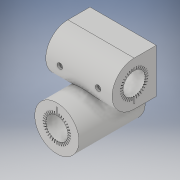
# Autodesk Inventor part: cam_holder_angle_part
Saved by Autodesk Inventor 2019 (Build 230136000, 136)
## iProperties
Created: 2024-08-06
Part Number: cam_holder_angle_part
Material: Generisch
Document SubType Name: Modeling
Designer: nic
Density: 1 g/cm^3
Appearance: Vorgabe
Author: nic
Autodesk Inventor part; units mm, degrees
ref_plane "YZ Plane" through (0, 0, 0) normal (1, 0, 0) x (0, 1, 0)
sketch "Skizze1" plane through (0, 0, 0) normal (0, 0, 1) x (1, 0, 0)
  circle A0 centre (0, 0) radius 10.05
  circle A1 centre (0, 0) radius 20
  dimension "d0" = 20.1
  dimension "d1" = 40
  constraints: 2 centre point, 2 coincident
  measures "d0" diameter of A0
  measures "d1" diameter of A1
extrude "Extrusion1" add sketch "Skizze1" along normal blind 60
sketch "Skizze2" plane through (0, 0, 0) normal (1, 0, 0) x (0, 1, 0)
  line L0 (10.05, 0) -> (10.05, 60) projected
  line L1 (-20, 0) -> (20, 0) projected
  line L2 (20, 0) -> (20, 60) projected
  circle A0 centre (30.05, 20) radius 10.05
  arc A1 (50.05, 20) -> (20, 37.2915) centre (30.05, 20) ccw
  line L3 (20, 0) -> (50.05, 0)
  line L4 (50.05, 0) -> (50.05, 20)
  line L5 (50.05, 0) -> (20, 0)
  line L6 (20, 0) -> (20, 2.7085)
  line L7 (50.05, 20) -> (50.05, 0)
  arc A2 (50.05, 20) -> (10.05, 20) centre (30.05, 20) ccw
  line L8 (50.05, 0) -> (10.05, 0)
  line L9 (10.05, 0) -> (10.05, 20)
  line L10 (50.05, 20) -> (50.05, 0)
  point P0 (0, 0)
  constraints: 16 end point, 5 point on circle, 3 centre point, 3 horizontal, 3 perpendicular, 3 tangent, 2 coincident, 2 parallel, 2 point on line
extrude "Extrusion2" add sketch "Skizze2" along normal blind 30 and the other way blind 30
sketch "Skizze3" plane through (30, 0, 0) normal (1, 0, 0) x (0, 0, -1)
  circle A0 centre (-20, 30.05) radius 10.05 construction
  line L0 (0, 10.05) -> (0, 50.05) construction
  line L1 (0, 50.05) -> (-20, 50.05) construction
  arc A1 (-20, 50.05) -> (-20, 10.05) centre (-20, 30.05) ccw construction
  line L2 (-20, 10.05) -> (0, 10.05) construction
  line L3 (-27.55, 30.3) -> (-32.55, 30.3)
  line L4 (-32.55, 30.3) -> (-32.55, 29.8)
  line L5 (-32.55, 29.8) -> (-27.55, 29.8)
  line L6 (-27.55, 29.8) -> (-27.55, 30.3)
  circle A2 centre (-20, 30.05) radius 10.05 projected
  line L7 (-27.55, 30.3) -> (-32.55, 29.8) construction
  line L8 (-32.55, 30.3) -> (-27.55, 29.8) construction
  line L9 (-27.4787, 28.9852) -> (-32.4027, 28.1169)
  line L10 (-32.4027, 28.1169) -> (-32.3159, 27.6245)
  line L11 (-32.3159, 27.6245) -> (-27.3919, 28.4928)
  line L12 (-27.3919, 28.4928) -> (-27.4787, 28.9852)
  line L13 (-27.4787, 28.9852) -> (-32.3159, 27.6245) construction
  line L14 (-32.4027, 28.1169) -> (-27.3919, 28.4928) construction
  line L15 (-27.1802, 27.7027) -> (-31.8786, 25.9926)
  line L16 (-31.8786, 25.9926) -> (-31.7076, 25.5227)
  line L17 (-31.7076, 25.5227) -> (-27.0092, 27.2328)
  line L18 (-27.0092, 27.2328) -> (-27.1802, 27.7027)
  line L19 (-27.1802, 27.7027) -> (-31.7076, 25.5227) construction
  line L20 (-31.8786, 25.9926) -> (-27.0092, 27.2328) construction
  line L21 (-26.6635, 26.4915) -> (-30.9936, 23.9915)
  line L22 (-30.9936, 23.9915) -> (-30.7436, 23.5585)
  line L23 (-30.7436, 23.5585) -> (-26.4135, 26.0585)
  line L24 (-26.4135, 26.0585) -> (-26.6635, 26.4915)
  line L25 (-26.6635, 26.4915) -> (-30.7436, 23.5585) construction
  line L26 (-30.9936, 23.9915) -> (-26.4135, 26.0585) construction
  line L27 (-25.9443, 25.3885) -> (-29.7746, 22.1745)
  line L28 (-29.7746, 22.1745) -> (-29.4532, 21.7915)
  line L29 (-29.4532, 21.7915) -> (-25.6229, 25.0054)
  line L30 (-25.6229, 25.0054) -> (-25.9443, 25.3885)
  line L31 (-25.9443, 25.3885) -> (-29.4532, 21.7915) construction
  line L32 (-29.7746, 22.1745) -> (-25.6229, 25.0054) construction
  line L33 (-25.0446, 24.4271) -> (-28.2585, 20.5968)
  line L34 (-28.2585, 20.5968) -> (-27.8755, 20.2754)
  line L35 (-27.8755, 20.2754) -> (-24.6615, 24.1057)
  line L36 (-24.6615, 24.1057) -> (-25.0446, 24.4271)
  line L37 (-25.0446, 24.4271) -> (-27.8755, 20.2754) construction
  line L38 (-28.2585, 20.5968) -> (-24.6615, 24.1057) construction
  line L39 (-23.9915, 23.6365) -> (-26.4915, 19.3064)
  line L40 (-26.4915, 19.3064) -> (-26.0585, 19.0564)
  line L41 (-26.0585, 19.0564) -> (-23.5585, 23.3865)
  line L42 (-23.5585, 23.3865) -> (-23.9915, 23.6365)
  line L43 (-23.9915, 23.6365) -> (-26.0585, 19.0564) construction
  line L44 (-26.4915, 19.3064) -> (-23.5585, 23.3865) construction
  line L45 (-22.8172, 23.0408) -> (-24.5273, 18.3424)
  line L46 (-24.5273, 18.3424) -> (-24.0574, 18.1714)
  line L47 (-24.0574, 18.1714) -> (-22.3473, 22.8698)
  line L48 (-22.3473, 22.8698) -> (-22.8172, 23.0408)
  line L49 (-22.8172, 23.0408) -> (-24.0574, 18.1714) construction
  line L50 (-24.5273, 18.3424) -> (-22.3473, 22.8698) construction
  line L51 (-21.5572, 22.6581) -> (-22.4255, 17.7341)
  line L52 (-22.4255, 17.7341) -> (-21.9331, 17.6473)
  line L53 (-21.9331, 17.6473) -> (-21.0648, 22.5713)
  line L54 (-21.0648, 22.5713) -> (-21.5572, 22.6581)
  line L55 (-21.5572, 22.6581) -> (-21.9331, 17.6473) construction
  line L56 (-22.4255, 17.7341) -> (-21.0648, 22.5713) construction
  line L57 (-20.25, 22.5) -> (-20.25, 17.5)
  line L58 (-20.25, 17.5) -> (-19.75, 17.5)
  line L59 (-19.75, 17.5) -> (-19.75, 22.5)
  line L60 (-19.75, 22.5) -> (-20.25, 22.5)
  line L61 (-20.25, 22.5) -> (-19.75, 17.5) construction
  line L62 (-20.25, 17.5) -> (-19.75, 22.5) construction
  line L63 (-18.9352, 22.5713) -> (-18.0669, 17.6473)
  line L64 (-18.0669, 17.6473) -> (-17.5745, 17.7341)
  line L65 (-17.5745, 17.7341) -> (-18.4428, 22.6581)
  line L66 (-18.4428, 22.6581) -> (-18.9352, 22.5713)
  line L67 (-18.9352, 22.5713) -> (-17.5745, 17.7341) construction
  line L68 (-18.0669, 17.6473) -> (-18.4428, 22.6581) construction
  line L69 (-17.6527, 22.8698) -> (-15.9426, 18.1714)
  line L70 (-15.9426, 18.1714) -> (-15.4727, 18.3424)
  line L71 (-15.4727, 18.3424) -> (-17.1828, 23.0408)
  line L72 (-17.1828, 23.0408) -> (-17.6527, 22.8698)
  line L73 (-17.6527, 22.8698) -> (-15.4727, 18.3424) construction
  line L74 (-15.9426, 18.1714) -> (-17.1828, 23.0408) construction
  line L75 (-16.4415, 23.3865) -> (-13.9415, 19.0564)
  line L76 (-13.9415, 19.0564) -> (-13.5085, 19.3064)
  line L77 (-13.5085, 19.3064) -> (-16.0085, 23.6365)
  line L78 (-16.0085, 23.6365) -> (-16.4415, 23.3865)
  line L79 (-16.4415, 23.3865) -> (-13.5085, 19.3064) construction
  line L80 (-13.9415, 19.0564) -> (-16.0085, 23.6365) construction
  line L81 (-15.3385, 24.1057) -> (-12.1245, 20.2754)
  line L82 (-12.1245, 20.2754) -> (-11.7415, 20.5968)
  line L83 (-11.7415, 20.5968) -> (-14.9554, 24.4271)
  line L84 (-14.9554, 24.4271) -> (-15.3385, 24.1057)
  line L85 (-15.3385, 24.1057) -> (-11.7415, 20.5968) construction
  line L86 (-12.1245, 20.2754) -> (-14.9554, 24.4271) construction
  line L87 (-14.3771, 25.0054) -> (-10.5468, 21.7915)
  line L88 (-10.5468, 21.7915) -> (-10.2254, 22.1745)
  line L89 (-10.2254, 22.1745) -> (-14.0557, 25.3885)
  line L90 (-14.0557, 25.3885) -> (-14.3771, 25.0054)
  line L91 (-14.3771, 25.0054) -> (-10.2254, 22.1745) construction
  line L92 (-10.5468, 21.7915) -> (-14.0557, 25.3885) construction
  line L93 (-13.5865, 26.0585) -> (-9.2564, 23.5585)
  line L94 (-9.2564, 23.5585) -> (-9.0064, 23.9915)
  line L95 (-9.0064, 23.9915) -> (-13.3365, 26.4915)
  line L96 (-13.3365, 26.4915) -> (-13.5865, 26.0585)
  line L97 (-13.5865, 26.0585) -> (-9.0064, 23.9915) construction
  line L98 (-9.2564, 23.5585) -> (-13.3365, 26.4915) construction
  line L99 (-12.9908, 27.2328) -> (-8.2924, 25.5227)
  line L100 (-8.2924, 25.5227) -> (-8.1214, 25.9926)
  line L101 (-8.1214, 25.9926) -> (-12.8198, 27.7027)
  line L102 (-12.8198, 27.7027) -> (-12.9908, 27.2328)
  line L103 (-12.9908, 27.2328) -> (-8.1214, 25.9926) construction
  line L104 (-8.2924, 25.5227) -> (-12.8198, 27.7027) construction
  line L105 (-12.6081, 28.4928) -> (-7.6841, 27.6245)
  line L106 (-7.6841, 27.6245) -> (-7.5973, 28.1169)
  line L107 (-7.5973, 28.1169) -> (-12.5213, 28.9852)
  line L108 (-12.5213, 28.9852) -> (-12.6081, 28.4928)
  line L109 (-12.6081, 28.4928) -> (-7.5973, 28.1169) construction
  line L110 (-7.6841, 27.6245) -> (-12.5213, 28.9852) construction
  line L111 (-12.45, 29.8) -> (-7.45, 29.8)
  line L112 (-7.45, 29.8) -> (-7.45, 30.3)
  line L113 (-7.45, 30.3) -> (-12.45, 30.3)
  line L114 (-12.45, 30.3) -> (-12.45, 29.8)
  line L115 (-12.45, 29.8) -> (-7.45, 30.3) construction
  line L116 (-7.45, 29.8) -> (-12.45, 30.3) construction
  line L117 (-12.5213, 31.1148) -> (-7.5973, 31.9831)
  line L118 (-7.5973, 31.9831) -> (-7.6841, 32.4755)
  line L119 (-7.6841, 32.4755) -> (-12.6081, 31.6072)
  line L120 (-12.6081, 31.6072) -> (-12.5213, 31.1148)
  line L121 (-12.5213, 31.1148) -> (-7.6841, 32.4755) construction
  line L122 (-7.5973, 31.9831) -> (-12.6081, 31.6072) construction
  line L123 (-12.8198, 32.3973) -> (-8.1214, 34.1074)
  line L124 (-8.1214, 34.1074) -> (-8.2924, 34.5773)
  line L125 (-8.2924, 34.5773) -> (-12.9908, 32.8672)
  line L126 (-12.9908, 32.8672) -> (-12.8198, 32.3973)
  line L127 (-12.8198, 32.3973) -> (-8.2924, 34.5773) construction
  line L128 (-8.1214, 34.1074) -> (-12.9908, 32.8672) construction
  line L129 (-13.3365, 33.6085) -> (-9.0064, 36.1085)
  line L130 (-9.0064, 36.1085) -> (-9.2564, 36.5415)
  line L131 (-9.2564, 36.5415) -> (-13.5865, 34.0415)
  line L132 (-13.5865, 34.0415) -> (-13.3365, 33.6085)
  line L133 (-13.3365, 33.6085) -> (-9.2564, 36.5415) construction
  line L134 (-9.0064, 36.1085) -> (-13.5865, 34.0415) construction
  line L135 (-14.0557, 34.7115) -> (-10.2254, 37.9255)
  line L136 (-10.2254, 37.9255) -> (-10.5468, 38.3085)
  line L137 (-10.5468, 38.3085) -> (-14.3771, 35.0946)
  line L138 (-14.3771, 35.0946) -> (-14.0557, 34.7115)
  line L139 (-14.0557, 34.7115) -> (-10.5468, 38.3085) construction
  line L140 (-10.2254, 37.9255) -> (-14.3771, 35.0946) construction
  line L141 (-14.9554, 35.6729) -> (-11.7415, 39.5032)
  line L142 (-11.7415, 39.5032) -> (-12.1245, 39.8246)
  line L143 (-12.1245, 39.8246) -> (-15.3385, 35.9943)
  line L144 (-15.3385, 35.9943) -> (-14.9554, 35.6729)
  line L145 (-14.9554, 35.6729) -> (-12.1245, 39.8246) construction
  line L146 (-11.7415, 39.5032) -> (-15.3385, 35.9943) construction
  line L147 (-16.0085, 36.4635) -> (-13.5085, 40.7936)
  line L148 (-13.5085, 40.7936) -> (-13.9415, 41.0436)
  line L149 (-13.9415, 41.0436) -> (-16.4415, 36.7135)
  line L150 (-16.4415, 36.7135) -> (-16.0085, 36.4635)
  line L151 (-16.0085, 36.4635) -> (-13.9415, 41.0436) construction
  line L152 (-13.5085, 40.7936) -> (-16.4415, 36.7135) construction
  line L153 (-17.1828, 37.0592) -> (-15.4727, 41.7576)
  line L154 (-15.4727, 41.7576) -> (-15.9426, 41.9286)
  line L155 (-15.9426, 41.9286) -> (-17.6527, 37.2302)
  line L156 (-17.6527, 37.2302) -> (-17.1828, 37.0592)
  line L157 (-17.1828, 37.0592) -> (-15.9426, 41.9286) construction
  line L158 (-15.4727, 41.7576) -> (-17.6527, 37.2302) construction
  line L159 (-18.4428, 37.4419) -> (-17.5745, 42.3659)
  line L160 (-17.5745, 42.3659) -> (-18.0669, 42.4527)
  line L161 (-18.0669, 42.4527) -> (-18.9352, 37.5287)
  line L162 (-18.9352, 37.5287) -> (-18.4428, 37.4419)
  line L163 (-18.4428, 37.4419) -> (-18.0669, 42.4527) construction
  line L164 (-17.5745, 42.3659) -> (-18.9352, 37.5287) construction
  line L165 (-19.75, 37.6) -> (-19.75, 42.6)
  line L166 (-19.75, 42.6) -> (-20.25, 42.6)
  line L167 (-20.25, 42.6) -> (-20.25, 37.6)
  line L168 (-20.25, 37.6) -> (-19.75, 37.6)
  line L169 (-19.75, 37.6) -> (-20.25, 42.6) construction
  line L170 (-19.75, 42.6) -> (-20.25, 37.6) construction
  line L171 (-21.0648, 37.5287) -> (-21.9331, 42.4527)
  line L172 (-21.9331, 42.4527) -> (-22.4255, 42.3659)
  line L173 (-22.4255, 42.3659) -> (-21.5572, 37.4419)
  line L174 (-21.5572, 37.4419) -> (-21.0648, 37.5287)
  line L175 (-21.0648, 37.5287) -> (-22.4255, 42.3659) construction
  line L176 (-21.9331, 42.4527) -> (-21.5572, 37.4419) construction
  line L177 (-22.3473, 37.2302) -> (-24.0574, 41.9286)
  line L178 (-24.0574, 41.9286) -> (-24.5273, 41.7576)
  line L179 (-24.5273, 41.7576) -> (-22.8172, 37.0592)
  line L180 (-22.8172, 37.0592) -> (-22.3473, 37.2302)
  line L181 (-22.3473, 37.2302) -> (-24.5273, 41.7576) construction
  line L182 (-24.0574, 41.9286) -> (-22.8172, 37.0592) construction
  line L183 (-23.5585, 36.7135) -> (-26.0585, 41.0436)
  line L184 (-26.0585, 41.0436) -> (-26.4915, 40.7936)
  line L185 (-26.4915, 40.7936) -> (-23.9915, 36.4635)
  line L186 (-23.9915, 36.4635) -> (-23.5585, 36.7135)
  line L187 (-23.5585, 36.7135) -> (-26.4915, 40.7936) construction
  line L188 (-26.0585, 41.0436) -> (-23.9915, 36.4635) construction
  line L189 (-24.6615, 35.9943) -> (-27.8755, 39.8246)
  line L190 (-27.8755, 39.8246) -> (-28.2585, 39.5032)
  line L191 (-28.2585, 39.5032) -> (-25.0446, 35.6729)
  line L192 (-25.0446, 35.6729) -> (-24.6615, 35.9943)
  line L193 (-24.6615, 35.9943) -> (-28.2585, 39.5032) construction
  line L194 (-27.8755, 39.8246) -> (-25.0446, 35.6729) construction
  line L195 (-25.6229, 35.0946) -> (-29.4532, 38.3085)
  line L196 (-29.4532, 38.3085) -> (-29.7746, 37.9255)
  line L197 (-29.7746, 37.9255) -> (-25.9443, 34.7115)
  line L198 (-25.9443, 34.7115) -> (-25.6229, 35.0946)
  line L199 (-25.6229, 35.0946) -> (-29.7746, 37.9255) construction
  line L200 (-29.4532, 38.3085) -> (-25.9443, 34.7115) construction
  line L201 (-26.4135, 34.0415) -> (-30.7436, 36.5415)
  line L202 (-30.7436, 36.5415) -> (-30.9936, 36.1085)
  line L203 (-30.9936, 36.1085) -> (-26.6635, 33.6085)
  line L204 (-26.6635, 33.6085) -> (-26.4135, 34.0415)
  line L205 (-26.4135, 34.0415) -> (-30.9936, 36.1085) construction
  line L206 (-30.7436, 36.5415) -> (-26.6635, 33.6085) construction
  line L207 (-27.0092, 32.8672) -> (-31.7076, 34.5773)
  line L208 (-31.7076, 34.5773) -> (-31.8786, 34.1074)
  line L209 (-31.8786, 34.1074) -> (-27.1802, 32.3973)
  line L210 (-27.1802, 32.3973) -> (-27.0092, 32.8672)
  line L211 (-27.0092, 32.8672) -> (-31.8786, 34.1074) construction
  line L212 (-31.7076, 34.5773) -> (-27.1802, 32.3973) construction
  line L213 (-27.3919, 31.6072) -> (-32.3159, 32.4755)
  line L214 (-32.3159, 32.4755) -> (-32.4027, 31.9831)
  line L215 (-32.4027, 31.9831) -> (-27.4787, 31.1148)
  line L216 (-27.4787, 31.1148) -> (-27.3919, 31.6072)
  line L217 (-27.3919, 31.6072) -> (-32.4027, 31.9831) construction
  line L218 (-32.3159, 32.4755) -> (-27.4787, 31.1148) construction
  line L219 (-19.75, 22.5) -> (-20.306, 22.5)
  line L220 (-20.306, 22.5) -> (-20.306, 14.42)
  line L221 (-20.306, 14.42) -> (-19.75, 14.42)
  line L222 (-19.75, 14.42) -> (-19.75, 22.5)
  point P0 (0, 0)
  point P1 (-30.05, 30.05)
  point P2 (-29.8973, 28.3048)
  point P3 (-29.4439, 26.6127)
  point P4 (-28.7036, 25.025)
  point P5 (-27.6987, 23.59)
  point P6 (-26.46, 22.3513)
  point P7 (-25.025, 21.3464)
  point P8 (-23.4373, 20.6061)
  point P9 (-21.7452, 20.1527)
  point P10 (-20, 20)
  point P11 (-18.2548, 20.1527)
  point P12 (-16.5627, 20.6061)
  point P13 (-14.975, 21.3464)
  point P14 (-13.54, 22.3513)
  point P15 (-12.3013, 23.59)
  point P16 (-11.2964, 25.025)
  point P17 (-10.5561, 26.6127)
  point P18 (-10.1027, 28.3048)
  point P19 (-9.95, 30.05)
  point P20 (-10.1027, 31.7952)
  point P21 (-10.5561, 33.4873)
  point P22 (-11.2964, 35.075)
  point P23 (-12.3013, 36.51)
  point P24 (-13.54, 37.7487)
  point P25 (-14.975, 38.7536)
  point P26 (-16.5627, 39.4939)
  point P27 (-18.2548, 39.9473)
  point P28 (-20, 40.1)
  point P29 (-21.7452, 39.9473)
  point P30 (-23.4373, 39.4939)
  point P31 (-25.025, 38.7536)
  point P32 (-26.46, 37.7487)
  point P33 (-27.6987, 36.51)
  point P34 (-28.7036, 35.075)
  point P35 (-29.4439, 33.4873)
  point P36 (-29.8973, 31.7952)
  dimension "d10" = 5
  dimension "d11" = 0.5
  dimension "d14" = 360
  constraints: 440 end point, 72 midpoint, 4 parallel, 2 horizontal, 2 perpendicular, 1 horizontal alignment, 398 other
  measures "d10" distance of L5.end L4.end
  measures "d11" distance of L4.end L3.end
extrude "Extrusion3" cut sketch "Skizze3" against normal blind 0.5 contours L6 L5 A2 L3 | A2 L5 L4 L3 | L215 L214 L213 A2 | A2 L213 L216 L215 | L9 L12 L11 A2 | A2 L11 L10 L9 | L209 L208 L207 A2 | A2 L207 L210 L209 | L15 L18 L17 A2 | A2 L17 L16 L15 | L203 L202 L201 A2 | A2 L201 L204 L203 | L21 L24 L23 A2 | A2 L23 L22 L21 | L197 L196 L195 A2 | A2 L195 L198 L197 | L27 L30 L29 A2 | A2 L29 L28 L27 | L191 L190 L189 A2 | A2 L189 L192 L191 | L33 L36 L35 A2 | A2 L35 L34 L33 | L185 L184 L183 A2 | A2 L183 L186 L185 | L39 L42 L41 A2 | A2 L41 L40 L39 | L179 L178 L177 A2 | A2 L177 L180 L179 | L45 L48 L47 A2 | A2 L47 L46 L45 | L173 L172 L171 A2 | A2 L171 L174 L173 | L51 L54 L53 A2 | A2 L53 L52 L51 | L167 L166 L165 A2 | A2 L165 L168 L167 | L220 L219 L57 A2 | A2 L57 L58 L222 L221 L220 | L161 L160 L159 A2 | A2 L159 L162 L161 | L57 L60 L59 A2 | A2 L59 L58 L57 | L155 L154 L153 A2 | A2 L153 L156 L155 | L63 L66 L65 A2 | A2 L65 L64 L63 | L149 L148 L147 A2 | A2 L147 L150 L149 | L69 L72 L71 A2 | A2 L71 L70 L69 | L143 L142 L141 A2 | A2 L141 L144 L143 | L75 L78 L77 A2 | A2 L77 L76 L75 | L137 L136 L135 A2 | A2 L135 L138 L137 | L81 L84 L83 A2 | A2 L83 L82 L81 | L131 L130 L129 A2 | A2 L129 L132 L131 | L87 L90 L89 A2 | A2 L89 L88 L87 | L125 L124 L123 A2 | A2 L123 L126 L125 | L93 L96 L95 A2 | A2 L95 L94 L93 | L119 L118 L117 A2 | A2 L117 L120 L119 | L99 L102 L101 A2 | A2 L101 L100 L99 | L113 L112 L111 A2 | A2 L111 L114 L113 | L105 L108 L107 A2 | A2 L107 L106 L105
sketch "Skizze4" plane through (0, 0, 60) normal (0, 0, 1) x (1, 0, 0)
  circle A0 centre (0, 0) radius 10.05 construction
  circle A1 centre (0, 0) radius 20 construction
  line L0 (0.25, 7.55) -> (-0.25, 7.55)
  line L1 (-0.25, 7.55) -> (-0.25, 12.55)
  line L2 (-0.25, 12.55) -> (0.25, 12.55)
  line L3 (0.25, 12.55) -> (0.25, 7.55)
  circle A2 centre (0, 0) radius 10.05 projected
  line L4 (0.25, 7.55) -> (-0.25, 12.55) construction
  line L5 (-0.25, 7.55) -> (0.25, 12.55) construction
  line L6 (-1.0648, 7.4787) -> (-1.5572, 7.3919)
  line L7 (-1.5572, 7.3919) -> (-2.4255, 12.3159)
  line L8 (-2.4255, 12.3159) -> (-1.9331, 12.4027)
  line L9 (-1.9331, 12.4027) -> (-1.0648, 7.4787)
  line L10 (-1.0648, 7.4787) -> (-2.4255, 12.3159) construction
  line L11 (-1.5572, 7.3919) -> (-1.9331, 12.4027) construction
  line L12 (-2.3473, 7.1802) -> (-2.8172, 7.0092)
  line L13 (-2.8172, 7.0092) -> (-4.5273, 11.7076)
  line L14 (-4.5273, 11.7076) -> (-4.0574, 11.8786)
  line L15 (-4.0574, 11.8786) -> (-2.3473, 7.1802)
  line L16 (-2.3473, 7.1802) -> (-4.5273, 11.7076) construction
  line L17 (-2.8172, 7.0092) -> (-4.0574, 11.8786) construction
  line L18 (-3.5585, 6.6635) -> (-3.9915, 6.4135)
  line L19 (-3.9915, 6.4135) -> (-6.4915, 10.7436)
  line L20 (-6.4915, 10.7436) -> (-6.0585, 10.9936)
  line L21 (-6.0585, 10.9936) -> (-3.5585, 6.6635)
  line L22 (-3.5585, 6.6635) -> (-6.4915, 10.7436) construction
  line L23 (-3.9915, 6.4135) -> (-6.0585, 10.9936) construction
  line L24 (-4.6615, 5.9443) -> (-5.0446, 5.6229)
  line L25 (-5.0446, 5.6229) -> (-8.2585, 9.4532)
  line L26 (-8.2585, 9.4532) -> (-7.8755, 9.7746)
  line L27 (-7.8755, 9.7746) -> (-4.6615, 5.9443)
  line L28 (-4.6615, 5.9443) -> (-8.2585, 9.4532) construction
  line L29 (-5.0446, 5.6229) -> (-7.8755, 9.7746) construction
  line L30 (-5.6229, 5.0446) -> (-5.9443, 4.6615)
  line L31 (-5.9443, 4.6615) -> (-9.7746, 7.8755)
  line L32 (-9.7746, 7.8755) -> (-9.4532, 8.2585)
  line L33 (-9.4532, 8.2585) -> (-5.6229, 5.0446)
  line L34 (-5.6229, 5.0446) -> (-9.7746, 7.8755) construction
  line L35 (-5.9443, 4.6615) -> (-9.4532, 8.2585) construction
  line L36 (-6.4135, 3.9915) -> (-6.6635, 3.5585)
  line L37 (-6.6635, 3.5585) -> (-10.9936, 6.0585)
  line L38 (-10.9936, 6.0585) -> (-10.7436, 6.4915)
  line L39 (-10.7436, 6.4915) -> (-6.4135, 3.9915)
  line L40 (-6.4135, 3.9915) -> (-10.9936, 6.0585) construction
  line L41 (-6.6635, 3.5585) -> (-10.7436, 6.4915) construction
  line L42 (-7.0092, 2.8172) -> (-7.1802, 2.3473)
  line L43 (-7.1802, 2.3473) -> (-11.8786, 4.0574)
  line L44 (-11.8786, 4.0574) -> (-11.7076, 4.5273)
  line L45 (-11.7076, 4.5273) -> (-7.0092, 2.8172)
  line L46 (-7.0092, 2.8172) -> (-11.8786, 4.0574) construction
  line L47 (-7.1802, 2.3473) -> (-11.7076, 4.5273) construction
  line L48 (-7.3919, 1.5572) -> (-7.4787, 1.0648)
  line L49 (-7.4787, 1.0648) -> (-12.4027, 1.9331)
  line L50 (-12.4027, 1.9331) -> (-12.3159, 2.4255)
  line L51 (-12.3159, 2.4255) -> (-7.3919, 1.5572)
  line L52 (-7.3919, 1.5572) -> (-12.4027, 1.9331) construction
  line L53 (-7.4787, 1.0648) -> (-12.3159, 2.4255) construction
  line L54 (-7.55, 0.25) -> (-7.55, -0.25)
  line L55 (-7.55, -0.25) -> (-12.55, -0.25)
  line L56 (-12.55, -0.25) -> (-12.55, 0.25)
  line L57 (-12.55, 0.25) -> (-7.55, 0.25)
  line L58 (-7.55, 0.25) -> (-12.55, -0.25) construction
  line L59 (-7.55, -0.25) -> (-12.55, 0.25) construction
  line L60 (-7.4787, -1.0648) -> (-7.3919, -1.5572)
  line L61 (-7.3919, -1.5572) -> (-12.3159, -2.4255)
  line L62 (-12.3159, -2.4255) -> (-12.4027, -1.9331)
  line L63 (-12.4027, -1.9331) -> (-7.4787, -1.0648)
  line L64 (-7.4787, -1.0648) -> (-12.3159, -2.4255) construction
  line L65 (-7.3919, -1.5572) -> (-12.4027, -1.9331) construction
  line L66 (-7.1802, -2.3473) -> (-7.0092, -2.8172)
  line L67 (-7.0092, -2.8172) -> (-11.7076, -4.5273)
  line L68 (-11.7076, -4.5273) -> (-11.8786, -4.0574)
  line L69 (-11.8786, -4.0574) -> (-7.1802, -2.3473)
  line L70 (-7.1802, -2.3473) -> (-11.7076, -4.5273) construction
  line L71 (-7.0092, -2.8172) -> (-11.8786, -4.0574) construction
  line L72 (-6.6635, -3.5585) -> (-6.4135, -3.9915)
  line L73 (-6.4135, -3.9915) -> (-10.7436, -6.4915)
  line L74 (-10.7436, -6.4915) -> (-10.9936, -6.0585)
  line L75 (-10.9936, -6.0585) -> (-6.6635, -3.5585)
  line L76 (-6.6635, -3.5585) -> (-10.7436, -6.4915) construction
  line L77 (-6.4135, -3.9915) -> (-10.9936, -6.0585) construction
  line L78 (-5.9443, -4.6615) -> (-5.6229, -5.0446)
  line L79 (-5.6229, -5.0446) -> (-9.4532, -8.2585)
  line L80 (-9.4532, -8.2585) -> (-9.7746, -7.8755)
  line L81 (-9.7746, -7.8755) -> (-5.9443, -4.6615)
  line L82 (-5.9443, -4.6615) -> (-9.4532, -8.2585) construction
  line L83 (-5.6229, -5.0446) -> (-9.7746, -7.8755) construction
  line L84 (-5.0446, -5.6229) -> (-4.6615, -5.9443)
  line L85 (-4.6615, -5.9443) -> (-7.8755, -9.7746)
  line L86 (-7.8755, -9.7746) -> (-8.2585, -9.4532)
  line L87 (-8.2585, -9.4532) -> (-5.0446, -5.6229)
  line L88 (-5.0446, -5.6229) -> (-7.8755, -9.7746) construction
  line L89 (-4.6615, -5.9443) -> (-8.2585, -9.4532) construction
  line L90 (-3.9915, -6.4135) -> (-3.5585, -6.6635)
  line L91 (-3.5585, -6.6635) -> (-6.0585, -10.9936)
  line L92 (-6.0585, -10.9936) -> (-6.4915, -10.7436)
  line L93 (-6.4915, -10.7436) -> (-3.9915, -6.4135)
  line L94 (-3.9915, -6.4135) -> (-6.0585, -10.9936) construction
  line L95 (-3.5585, -6.6635) -> (-6.4915, -10.7436) construction
  line L96 (-2.8172, -7.0092) -> (-2.3473, -7.1802)
  line L97 (-2.3473, -7.1802) -> (-4.0574, -11.8786)
  line L98 (-4.0574, -11.8786) -> (-4.5273, -11.7076)
  line L99 (-4.5273, -11.7076) -> (-2.8172, -7.0092)
  line L100 (-2.8172, -7.0092) -> (-4.0574, -11.8786) construction
  line L101 (-2.3473, -7.1802) -> (-4.5273, -11.7076) construction
  line L102 (-1.5572, -7.3919) -> (-1.0648, -7.4787)
  line L103 (-1.0648, -7.4787) -> (-1.9331, -12.4027)
  line L104 (-1.9331, -12.4027) -> (-2.4255, -12.3159)
  line L105 (-2.4255, -12.3159) -> (-1.5572, -7.3919)
  line L106 (-1.5572, -7.3919) -> (-1.9331, -12.4027) construction
  line L107 (-1.0648, -7.4787) -> (-2.4255, -12.3159) construction
  line L108 (-0.25, -7.55) -> (0.25, -7.55)
  line L109 (0.25, -7.55) -> (0.25, -12.55)
  line L110 (0.25, -12.55) -> (-0.25, -12.55)
  line L111 (-0.25, -12.55) -> (-0.25, -7.55)
  line L112 (-0.25, -7.55) -> (0.25, -12.55) construction
  line L113 (0.25, -7.55) -> (-0.25, -12.55) construction
  line L114 (1.0648, -7.4787) -> (1.5572, -7.3919)
  line L115 (1.5572, -7.3919) -> (2.4255, -12.3159)
  line L116 (2.4255, -12.3159) -> (1.9331, -12.4027)
  line L117 (1.9331, -12.4027) -> (1.0648, -7.4787)
  line L118 (1.0648, -7.4787) -> (2.4255, -12.3159) construction
  line L119 (1.5572, -7.3919) -> (1.9331, -12.4027) construction
  line L120 (2.3473, -7.1802) -> (2.8172, -7.0092)
  line L121 (2.8172, -7.0092) -> (4.5273, -11.7076)
  line L122 (4.5273, -11.7076) -> (4.0574, -11.8786)
  line L123 (4.0574, -11.8786) -> (2.3473, -7.1802)
  line L124 (2.3473, -7.1802) -> (4.5273, -11.7076) construction
  line L125 (2.8172, -7.0092) -> (4.0574, -11.8786) construction
  line L126 (3.5585, -6.6635) -> (3.9915, -6.4135)
  line L127 (3.9915, -6.4135) -> (6.4915, -10.7436)
  line L128 (6.4915, -10.7436) -> (6.0585, -10.9936)
  line L129 (6.0585, -10.9936) -> (3.5585, -6.6635)
  line L130 (3.5585, -6.6635) -> (6.4915, -10.7436) construction
  line L131 (3.9915, -6.4135) -> (6.0585, -10.9936) construction
  line L132 (4.6615, -5.9443) -> (5.0446, -5.6229)
  line L133 (5.0446, -5.6229) -> (8.2585, -9.4532)
  line L134 (8.2585, -9.4532) -> (7.8755, -9.7746)
  line L135 (7.8755, -9.7746) -> (4.6615, -5.9443)
  line L136 (4.6615, -5.9443) -> (8.2585, -9.4532) construction
  line L137 (5.0446, -5.6229) -> (7.8755, -9.7746) construction
  line L138 (5.6229, -5.0446) -> (5.9443, -4.6615)
  line L139 (5.9443, -4.6615) -> (9.7746, -7.8755)
  line L140 (9.7746, -7.8755) -> (9.4532, -8.2585)
  line L141 (9.4532, -8.2585) -> (5.6229, -5.0446)
  line L142 (5.6229, -5.0446) -> (9.7746, -7.8755) construction
  line L143 (5.9443, -4.6615) -> (9.4532, -8.2585) construction
  line L144 (6.4135, -3.9915) -> (6.6635, -3.5585)
  line L145 (6.6635, -3.5585) -> (10.9936, -6.0585)
  line L146 (10.9936, -6.0585) -> (10.7436, -6.4915)
  line L147 (10.7436, -6.4915) -> (6.4135, -3.9915)
  line L148 (6.4135, -3.9915) -> (10.9936, -6.0585) construction
  line L149 (6.6635, -3.5585) -> (10.7436, -6.4915) construction
  line L150 (7.0092, -2.8172) -> (7.1802, -2.3473)
  line L151 (7.1802, -2.3473) -> (11.8786, -4.0574)
  line L152 (11.8786, -4.0574) -> (11.7076, -4.5273)
  line L153 (11.7076, -4.5273) -> (7.0092, -2.8172)
  line L154 (7.0092, -2.8172) -> (11.8786, -4.0574) construction
  line L155 (7.1802, -2.3473) -> (11.7076, -4.5273) construction
  line L156 (7.3919, -1.5572) -> (7.4787, -1.0648)
  line L157 (7.4787, -1.0648) -> (12.4027, -1.9331)
  line L158 (12.4027, -1.9331) -> (12.3159, -2.4255)
  line L159 (12.3159, -2.4255) -> (7.3919, -1.5572)
  line L160 (7.3919, -1.5572) -> (12.4027, -1.9331) construction
  line L161 (7.4787, -1.0648) -> (12.3159, -2.4255) construction
  line L162 (7.55, -0.25) -> (7.55, 0.25)
  line L163 (7.55, 0.25) -> (12.55, 0.25)
  line L164 (12.55, 0.25) -> (12.55, -0.25)
  line L165 (12.55, -0.25) -> (7.55, -0.25)
  line L166 (7.55, -0.25) -> (12.55, 0.25) construction
  line L167 (7.55, 0.25) -> (12.55, -0.25) construction
  line L168 (7.4787, 1.0648) -> (7.3919, 1.5572)
  line L169 (7.3919, 1.5572) -> (12.3159, 2.4255)
  line L170 (12.3159, 2.4255) -> (12.4027, 1.9331)
  line L171 (12.4027, 1.9331) -> (7.4787, 1.0648)
  line L172 (7.4787, 1.0648) -> (12.3159, 2.4255) construction
  line L173 (7.3919, 1.5572) -> (12.4027, 1.9331) construction
  line L174 (7.1802, 2.3473) -> (7.0092, 2.8172)
  line L175 (7.0092, 2.8172) -> (11.7076, 4.5273)
  line L176 (11.7076, 4.5273) -> (11.8786, 4.0574)
  line L177 (11.8786, 4.0574) -> (7.1802, 2.3473)
  line L178 (7.1802, 2.3473) -> (11.7076, 4.5273) construction
  line L179 (7.0092, 2.8172) -> (11.8786, 4.0574) construction
  line L180 (6.6635, 3.5585) -> (6.4135, 3.9915)
  line L181 (6.4135, 3.9915) -> (10.7436, 6.4915)
  line L182 (10.7436, 6.4915) -> (10.9936, 6.0585)
  line L183 (10.9936, 6.0585) -> (6.6635, 3.5585)
  line L184 (6.6635, 3.5585) -> (10.7436, 6.4915) construction
  line L185 (6.4135, 3.9915) -> (10.9936, 6.0585) construction
  line L186 (5.9443, 4.6615) -> (5.6229, 5.0446)
  line L187 (5.6229, 5.0446) -> (9.4532, 8.2585)
  line L188 (9.4532, 8.2585) -> (9.7746, 7.8755)
  line L189 (9.7746, 7.8755) -> (5.9443, 4.6615)
  line L190 (5.9443, 4.6615) -> (9.4532, 8.2585) construction
  line L191 (5.6229, 5.0446) -> (9.7746, 7.8755) construction
  line L192 (5.0446, 5.6229) -> (4.6615, 5.9443)
  line L193 (4.6615, 5.9443) -> (7.8755, 9.7746)
  line L194 (7.8755, 9.7746) -> (8.2585, 9.4532)
  line L195 (8.2585, 9.4532) -> (5.0446, 5.6229)
  line L196 (5.0446, 5.6229) -> (7.8755, 9.7746) construction
  line L197 (4.6615, 5.9443) -> (8.2585, 9.4532) construction
  line L198 (3.9915, 6.4135) -> (3.5585, 6.6635)
  line L199 (3.5585, 6.6635) -> (6.0585, 10.9936)
  line L200 (6.0585, 10.9936) -> (6.4915, 10.7436)
  line L201 (6.4915, 10.7436) -> (3.9915, 6.4135)
  line L202 (3.9915, 6.4135) -> (6.0585, 10.9936) construction
  line L203 (3.5585, 6.6635) -> (6.4915, 10.7436) construction
  line L204 (2.8172, 7.0092) -> (2.3473, 7.1802)
  line L205 (2.3473, 7.1802) -> (4.0574, 11.8786)
  line L206 (4.0574, 11.8786) -> (4.5273, 11.7076)
  line L207 (4.5273, 11.7076) -> (2.8172, 7.0092)
  line L208 (2.8172, 7.0092) -> (4.0574, 11.8786) construction
  line L209 (2.3473, 7.1802) -> (4.5273, 11.7076) construction
  line L210 (1.5572, 7.3919) -> (1.0648, 7.4787)
  line L211 (1.0648, 7.4787) -> (1.9331, 12.4027)
  line L212 (1.9331, 12.4027) -> (2.4255, 12.3159)
  line L213 (2.4255, 12.3159) -> (1.5572, 7.3919)
  line L214 (1.5572, 7.3919) -> (1.9331, 12.4027) construction
  line L215 (1.0648, 7.4787) -> (2.4255, 12.3159) construction
  line L216 (-0.25, 3.3152) -> (0.25, 3.3152)
  line L217 (0.25, 3.3152) -> (0.25, 16.7848)
  line L218 (0.25, 16.7848) -> (-0.25, 16.7848)
  line L219 (-0.25, 16.7848) -> (-0.25, 3.3152)
  line L220 (-0.25, 3.3152) -> (0.25, 16.7848) construction
  line L221 (0.25, 3.3152) -> (-0.25, 16.7848) construction
  point P0 (0, 10.05)
  point P1 (-1.7452, 9.8973)
  point P2 (-3.4373, 9.4439)
  point P3 (-5.025, 8.7036)
  point P4 (-6.46, 7.6987)
  point P5 (-7.6987, 6.46)
  point P6 (-8.7036, 5.025)
  point P7 (-9.4439, 3.4373)
  point P8 (-9.8973, 1.7452)
  point P9 (-10.05, 0)
  point P10 (-9.8973, -1.7452)
  point P11 (-9.4439, -3.4373)
  point P12 (-8.7036, -5.025)
  point P13 (-7.6987, -6.46)
  point P14 (-6.46, -7.6987)
  point P15 (-5.025, -8.7036)
  point P16 (-3.4373, -9.4439)
  point P17 (-1.7452, -9.8973)
  point P18 (0, -10.05)
  point P19 (1.7452, -9.8973)
  point P20 (3.4373, -9.4439)
  point P21 (5.025, -8.7036)
  point P22 (6.46, -7.6987)
  point P23 (7.6987, -6.46)
  point P24 (8.7036, -5.025)
  point P25 (9.4439, -3.4373)
  point P26 (9.8973, -1.7452)
  point P27 (10.05, 0)
  point P28 (9.8973, 1.7452)
  point P29 (9.4439, 3.4373)
  point P30 (8.7036, 5.025)
  point P31 (7.6987, 6.46)
  point P32 (6.46, 7.6987)
  point P33 (5.025, 8.7036)
  point P34 (3.4373, 9.4439)
  point P35 (1.7452, 9.8973)
  dimension "d18" = 0.5
  dimension "d19" = 5
  dimension "d22" = 360
  constraints: 444 end point, 74 midpoint, 4 parallel, 2 horizontal, 2 perpendicular, 1 point on line, 1 vertical alignment, 398 other
  measures "d18" distance of L1.end L2.end
  measures "d19" distance of L0.end L1.end
extrude "Extrusion4" cut sketch "Skizze4" against normal blind 0.5 contours L217 L216 L219 L0 | L0 L1 A2 L3 | A2 L1 L2 L3 | L2 L219 L218 L217 | L211 L212 L213 A2 | A2 L213 L210 L211 | L9 L6 L7 A2 | A2 L7 L8 L9 | L205 L206 L207 A2 | A2 L207 L204 L205 | L15 L12 L13 A2 | A2 L13 L14 L15 | L199 L200 L201 A2 | A2 L201 L198 L199 | L21 L18 L19 A2 | A2 L19 L20 L21 | L193 L194 L195 A2 | A2 L195 L192 L193 | L27 L24 L25 A2 | A2 L25 L26 L27 | L187 L188 L189 A2 | A2 L189 L186 L187 | L33 L30 L31 A2 | A2 L31 L32 L33 | L181 L182 L183 A2 | A2 L183 L180 L181 | L39 L36 L37 A2 | A2 L37 L38 L39 | L175 L176 L177 A2 | A2 L177 L174 L175 | L45 L42 L43 A2 | A2 L43 L44 L45 | L169 L170 L171 A2 | A2 L171 L168 L169 | L51 L48 L49 A2 | A2 L49 L50 L51 | L163 L164 L165 A2 | A2 L165 L162 L163 | L57 L54 L55 A2 | A2 L55 L56 L57 | L63 L60 L61 A2 | A2 L61 L62 L63 | L157 L158 L159 A2 | A2 L159 L156 L157 | L69 L66 L67 A2 | A2 L67 L68 L69 | L151 L152 L153 A2 | A2 L153 L150 L151 | L75 L72 L73 A2 | A2 L73 L74 L75 | L145 L146 L147 A2 | A2 L147 L144 L145 | L81 L78 L79 A2 | A2 L79 L80 L81 | L139 L140 L141 A2 | A2 L141 L138 L139 | L87 L84 L85 A2 | A2 L85 L86 L87 | L133 L134 L135 A2 | A2 L135 L132 L133 | L93 L90 L91 A2 | A2 L91 L92 L93 | L127 L128 L129 A2 | A2 L129 L126 L127 | L99 L96 L97 A2 | A2 L97 L98 L99 | L121 L122 L123 A2 | A2 L123 L120 L121 | L105 L102 L103 A2 | A2 L103 L104 L105 | L115 L116 L117 A2 | A2 L117 L114 L115 | L111 L108 L109 A2 | A2 L109 L110 L111
ref_plane "Arbeitsebene1" through (0, -20, 0) normal (0, 1, 0) x (-1, 0, 0)
sketch "Skizze5" plane through (0, -20, 0) normal (0, 1, 0) x (-1, 0, 0)
  line L0 (17.2915, 20) -> (17.2915, 0) projected
  line L1 (-17.2915, 0) -> (17.2915, 0) projected
  line L2 (-17.2915, 0) -> (-17.2915, 20) projected
  line L3 (20, 60) -> (-20, 60) projected
  line L4 (0, 0) -> (0, 60)
  point P0 (0, 15.4815)
  point P1 (0, 44.9369)
  constraints: 2 end point, 2 point on line, 1 horizontal alignment, 1 midpoint
hole "Bohrung1" at (0, -20, 15.4815) at (0, -20, 44.9369) direction (0, 1, 0) diameter 3.8 depth 11 tip angle 118 counterbore diameter 5 counterbore depth 2
ref_plane "Arbeitsebene2" through (0, 0, 40) normal (0, 0, 1) x (1, 0, 0)
sketch "Skizze6" plane through (0, 0, 40) normal (0, 0, 1) x (1, 0, 0)
  line L0 (17.2915, 10.05) -> (30, 10.05) projected
  line L1 (30, 50.05) -> (30, 50.05) projected
  line L2 (-30, 50.05) -> (30, 50.05) projected
  line L3 (-30, 10.05) -> (-30, 50.05) projected
  line L4 (-30, 10.05) -> (-17.2915, 10.05) projected
  line L5 (-30, 20) -> (-30, 40.1) projected
  line L6 (-30, 30.05) -> (30, 30.05)
  line L7 (30, 50.05) -> (30, 50.05) projected
  point P0 (0, 0)
  point P1 (-17.2915, 30.05)
  point P2 (17.2915, 30.05)
  constraints: 3 point on line, 2 end point, 1 horizontal alignment, 1 midpoint
hole "Bohrung2" at (-17.2915, 30.05, 40) at (17.2915, 30.05, 40) direction (0, 0, -1) diameter 3.8 depth 11 tip angle 118 counterbore diameter 5 counterbore depth 2
